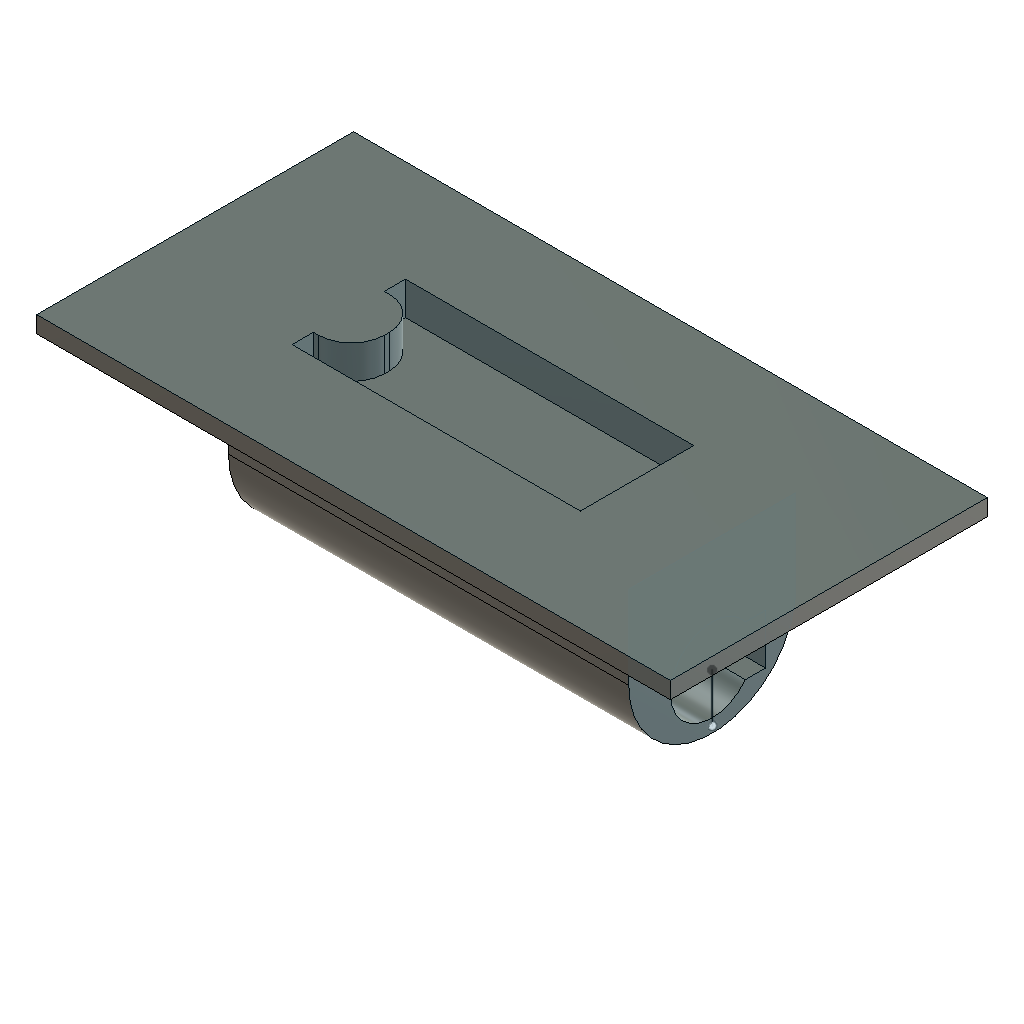
balancin (Ensamblaje) (Autodesk Fusion 360 archive; units mm, degrees)
design "balancin"
part number: 2026-09-28-04-10-51-977
Autodesk Fusion 360 part; units mm, degrees
sketch "Boceto1" plane through (0, 0, 0) normal (0, 1, 0) x (1, 0, 0)
  line L0 (-30, 20) -> (160, 20)
  line L1 (160, 20) -> (160, -75)
  line L2 (160, -75) -> (-30, -75)
  line L3 (-30, -75) -> (-30, 20)
  dimension "d1" = 190
  dimension "d2" = 95
  constraint horizontal L0
  constraint vertical L1
  constraint horizontal L2
  constraint vertical L3
  measures "d1" distance of L0.start L0.end
  measures "d2" distance of L0.start L2.end
extrude "Extruir1" add sketch "Boceto1" along normal blind 5
sketch "Boceto2" plane through (0, 0, 0) normal (0, -1, 0) x (1, 0, 0)
  line L0 (160, 75) -> (-30, 75)
  line L1 (-30, 75) -> (-30, -20)
  line L2 (-30, -20) -> (160, -20)
  line L3 (160, -20) -> (160, 75)
  line L4 (-30, 27.5) -> (5, 27.5)
  line L5 (65, 52.5) -> (5, 52.5)
  line L6 (125, 27.5) -> (125, 2.5)
  line L7 (5, 52.5) -> (125, 52.5)
  line L8 (125, 52.5) -> (125, 2.5)
  line L9 (125, 2.5) -> (5, 2.5)
  line L10 (5, 2.5) -> (5, 52.5)
  point P0 (65, 27.5)
  dimension "d5" = 47.5
  dimension "d6" = 95
  dimension "d7" = 25
  dimension "d8" = 60
  dimension "d9" = 60
  dimension "d10" = 25
  constraint horizontal L7
  constraint vertical L8
  constraint horizontal L9
  constraint vertical L10
  constraint coincident L10 L4.end
  measures "d5" distance of L0.end L4.start
  measures "d6" distance of L4.start P0
  measures "d7" distance of L5.start P0
  measures "d8" distance of L5.start L5.end
  measures "d9" distance of L6.start P0
  measures "d10" distance of L6.start L6.end
extrude "Extruir2" add sketch "Boceto2" along normal blind 50 contours L5 L6 L7 L8 L9 L10
sketch "Boceto3" plane through (125, 0, 0) normal (1, 0, 0) x (0, 0, -1)
  line L0 (-2.5, 0) -> (-52.5, 0)
  line L1 (-52.5, 0) -> (-52.5, -50)
  line L2 (-52.5, -50) -> (-2.5, -50)
  line L3 (-2.5, -50) -> (-2.5, 0)
  line L4 (-52.5, -50) -> (-27.5, -50)
  line L5 (-27.5, -50) -> (-27.5, -46)
  circle A0 centre (-27.5, -33.525) radius 12.475
  dimension "d13" = 25
  dimension "d14" = 4
  dimension "d15" = 24.95
  constraint coincident L1.end L2.start
  constraint perpendicular L1 L4
  constraint perpendicular L4 L5
  constraint coincident L5.end A0
  measures "d13" distance of L1.end L4.end
  measures "d14" distance of L4.end L5.end
  measures "d15" diameter of A0
extrude "Extruir3" cut sketch "Boceto3" against normal blind 150 contours A0
sketch "Boceto4" plane through (125, 0, 0) normal (1, 0, 0) x (0, 0, -1)
  circle A0 centre (-27.5, -33.525) radius 12.475
  line L0 (-2.5, 0) -> (-52.5, 0)
  line L1 (-52.5, 0) -> (-52.5, -50)
  line L2 (-52.5, -50) -> (-2.5, -50)
  line L3 (-2.5, -50) -> (-2.5, 0)
  line L4 (-27.5, -33.525) -> (-18.5, -33.525)
  line L5 (-18.5, -33.525) -> (-18.5, -26.025)
  line L6 (-18.5, -26.025) -> (-11.5, -26.025)
  line L7 (-11.5, -26.025) -> (-11.5, -41.025)
  line L8 (-11.5, -41.025) -> (-18.5, -41.025)
  line L9 (-18.5, -41.025) -> (-18.5, -26.025)
  dimension "d18" = 9
  dimension "d19" = 7.5
  dimension "d20" = 7
  dimension "d21" = 15
  constraint coincident A0.centre L4.start
  constraint perpendicular L4 L5
  constraint horizontal L6
  constraint vertical L7
  constraint horizontal L8
  constraint vertical L9
  measures "d18" distance of A0.centre L4.end
  measures "d19" distance of L4.end L5.end
  measures "d20" distance of L5.end L6.end
  measures "d21" distance of L6.end L7.end
extrude "Extruir4" cut sketch "Boceto4" against normal blind 180 contours A0 L6 L7 L8
fillet "Empalme1" radius 25 2 edges at (65, -50, 2.5) (65, -50, 52.5)
sketch "Boceto5" plane through (0, 0, 0) normal (0, 0, 1) x (1, 0, 0)
  line L0 (64.5, -25) -> (64.5, -45)
  line L1 (68.5, -25) -> (68.5, -45)
  line L2 (65.5, -25) -> (65.5, -5)
  line L3 (64.5, -5) -> (64.5, -25)
  line L4 (64.5, -45) -> (54.5, -45)
  line L5 (54.5, -45) -> (64.5, -45)
  line L6 (64.5, -45) -> (64.5, -5)
  line L7 (64.5, -5) -> (54.5, -5)
  line L8 (54.5, -5) -> (54.5, -45)
  line L9 (68.5, -45) -> (75.5, -45)
  line L10 (75.5, -45) -> (65.5, -45)
  line L11 (65.5, -45) -> (65.5, -5)
  line L12 (65.5, -5) -> (75.5, -5)
  line L13 (75.5, -5) -> (75.5, -45)
  line L14 (54.5, -40.8747) -> (75.5, -40.8747)
  line L15 (54.5, -23.0491) -> (75.5, -23.0491)
  dimension "d33" = 20
  dimension "d35" = 20
  dimension "d36" = 10
  dimension "d37" = 7
  dimension "d38" = 10
  constraint vertical L2
  constraint vertical L3
  constraint perpendicular L0 L4
  constraint horizontal L5
  constraint vertical L6
  constraint horizontal L7
  constraint vertical L8
  constraint perpendicular L1 L9
  constraint horizontal L10
  constraint vertical L11
  constraint horizontal L12
  constraint vertical L13
  constraint coincident L8 L14.start
  constraint coincident L13 L14.end
  constraint perpendicular L13 L14
  constraint coincident L8 L15.start
  constraint coincident L13 L15.end
  constraint perpendicular L13 L15
  measures "d33" distance of L0.start L0.end
  measures "d35" distance of L0.start L3.start
  measures "d36" distance of L0.end L4.end
  measures "d37" distance of L1.end L9.end
  measures "d38" distance of L2.end L12.end
extrude "Extruir5" cut sketch "Boceto5" along normal blind 31 contours L0 L3 L6 L8 L14 L15 | L2 L11 L13 L14 L15
sketch "Boceto6" plane through (0, 0, 11.5) normal (0, 0, 1) x (1, 0, 0)
  line L0 (54.5, -40.8747) -> (54.5, -26.025)
  line L1 (54.5, -26.025) -> (5, -26.025)
  line L2 (5, -26.025) -> (5, -41.025)
  line L3 (5, -41.025) -> (125, -41.025)
  line L4 (125, -41.025) -> (125, -26.025)
  line L5 (125, -26.025) -> (75.5, -26.025)
  line L6 (75.5, -26.025) -> (75.5, -40.8747)
  line L7 (75.5, -40.8747) -> (65.5, -40.8747)
  line L8 (65.5, -40.8747) -> (65.5, -26.025)
  line L9 (65.5, -26.025) -> (64.5, -26.025)
  line L10 (64.5, -26.025) -> (64.5, -40.8747)
  line L11 (64.5, -40.8747) -> (54.5, -40.8747)
  line L12 (64.5, -48.0409) -> (65.5441, -48.0409)
  line L13 (65.5441, -48.0409) -> (65.5441, -10.5894)
  line L14 (65.5441, -10.5894) -> (64.5, -10.5894)
  line L15 (64.5, -10.5894) -> (64.5, -48.0409)
  constraint horizontal L12
  constraint vertical L13
  constraint horizontal L14
  constraint vertical L15
extrude "Extruir6" add sketch "Boceto6" along normal blind 30 contours L3 L7 L8 L9 L10 L13 L15 | L7 L8 L9 L13 L14 L15 | L3 L12 L13 L15
sketch "Boceto7" plane through (65.5441, 0, 0) normal (1, 0, 0) x (0, 0, -1)
  arc A0 (-17.7987, -48.0409) -> (-11.5, -44.2094) centre (-27.5, -25) ccw
  line L0 (-17.7987, -48.0409) -> (-11.5, -48.0409)
  line L1 (-11.5, -48.0409) -> (-11.5, -44.2094)
  arc A1 (-41.5, -45.7123) -> (-37.2013, -48.0409) centre (-27.5, -25) ccw
  line L2 (-41.5, -45.7123) -> (-41.5, -48.0409)
  line L3 (-41.5, -48.0409) -> (-37.2013, -48.0409)
extrude "Extruir7" cut sketch "Boceto7" against normal blind 9
sketch "Boceto8" plane through (125, 0, 0) normal (1, 0, 0) x (0, 0, -1)
  line L0 (-11.5, -41.025) -> (-17.5313, -41.025)
  arc A0 (-17.5313, -26.025) -> (-17.5313, -41.025) centre (-27.5, -33.525) ccw
  line L1 (-17.5313, -26.025) -> (-11.5, -26.025)
  line L2 (-11.5, -26.025) -> (-11.5, -41.025)
  arc A1 (-52.5, -25) -> (-2.5, -25) centre (-27.5, -25) ccw
  line L3 (-2.5, -25) -> (-2.5, 0)
  line L4 (-2.5, 0) -> (-52.5, 0)
  line L5 (-52.5, 0) -> (-52.5, -25)
  line L6 (-27.5, -33.525) -> (-27.5, -48)
  constraint coincident A0.centre L6.start
  constraint vertical L6
sketch "Boceto9" plane through (0, 5, 0) normal (0, 1, 0) x (-1, 0, 0)
  line L0 (30, 75) -> (-160, 75)
  line L1 (-160, 75) -> (-160, -20)
  line L2 (-160, -20) -> (30, -20)
  line L3 (30, -20) -> (30, 75)
  line L4 (30, 75) -> (30, 27.5)
  line L5 (30, 27.5) -> (-65, 27.5)
  line L6 (-65, 27.5) -> (-102.5, 27.5)
  line L7 (-102.5, 27.5) -> (-102.5, 44.5)
  line L8 (-102.5, 44.5) -> (-27.5, 44.5)
  line L9 (-27.5, 44.5) -> (-27.5, 10.5)
  line L10 (-27.5, 10.5) -> (-102.5, 10.5)
  line L11 (-102.5, 10.5) -> (-102.5, 44.5)
  dimension "d47" = 47.5
  dimension "d48" = 95
  dimension "d49" = 37.5
  dimension "d50" = 17
  dimension "d51" = 34
  dimension "d52" = 75
  constraint coincident L0.start L3.end
  constraint perpendicular L0 L4
  constraint perpendicular L4 L5
  constraint parallel L5 L6
  constraint perpendicular L6 L7
  constraint horizontal L8
  constraint vertical L9
  constraint horizontal L10
  constraint vertical L11
  measures "d47" distance of L0.start L4.end
  measures "d48" distance of L4.end L5.end
  measures "d49" distance of L5.end L6.end
  measures "d50" distance of L6.end L7.end
  measures "d51" distance of L7.end L10.end
  measures "d52" distance of L7.end L8.end
extrude "Extruir8" cut sketch "Boceto9" against normal blind 10 contours L5 L6 L9 L10 L11 | L5 L6 L7 L8 L9 L11
sketch "Boceto10" plane through (0, 5, 0) normal (0, 1, 0) x (-1, 0, 0)
  line L0 (-27.5, 44.5) -> (-27.5, 10.5)
  line L1 (-27.5, 10.5) -> (-102.5, 10.5)
  line L2 (-102.5, 10.5) -> (-102.5, 44.5)
  line L3 (-102.5, 44.5) -> (-27.5, 44.5)
  line L4 (30, 75) -> (-160, 75)
  line L5 (-160, 75) -> (-160, -20)
  line L6 (-160, -20) -> (30, -20)
  line L7 (30, -20) -> (30, 75)
  line L8 (-27.5, 44.5) -> (-16.0562, 44.5)
  line L9 (-16.0562, 44.5) -> (-16.0562, 38.0888)
  line L10 (-16.0562, 38.0888) -> (-27.5, 38.0888)
  line L11 (-27.5, 38.0888) -> (-27.5, 44.5)
  line L12 (-27.5, 10.5) -> (-16.0562, 10.5)
  line L13 (-16.0562, 10.5) -> (-16.0562, 16.8458)
  line L14 (-16.0562, 16.8458) -> (-27.5, 16.8458)
  line L15 (-27.5, 16.8458) -> (-27.5, 10.5)
  constraint horizontal L8
  constraint vertical L9
  constraint horizontal L10
  constraint vertical L11
  constraint coincident L0.start L3.end
  constraint horizontal L12
  constraint vertical L13
  constraint horizontal L14
  constraint vertical L15
  constraint coincident L0.end L1.start
extrude "Extruir9" cut sketch "Boceto10" against normal blind 10 contours L0 L8 L9 L10 L11 | L0 L12 L13 L14 L15
fillet "Empalme2" radius 10 2 edges at (27.5, 0, 16.8458) (27.5, 0, 38.0888)
sketch "Boceto11" plane through (0, 5, 0) normal (0, 1, 0) x (-1, 0, 0)
  arc A0 (-17.5, 38.0888) -> (-27.5, 28.0888) centre (-17.5, 28.0888) ccw
  line L0 (-27.5, 28.0888) -> (-27.5, 26.8458)
  arc A1 (-27.5, 26.8458) -> (-17.5, 16.8458) centre (-17.5, 26.8458) ccw
  line L1 (-17.5, 16.8458) -> (-16.0562, 16.8458)
  line L2 (-16.0562, 16.8458) -> (-16.0562, 10.5)
  line L3 (-16.0562, 10.5) -> (-102.5, 10.5)
  line L4 (-102.5, 10.5) -> (-102.5, 44.5)
  line L5 (-102.5, 44.5) -> (-16.0562, 44.5)
  line L6 (-16.0562, 44.5) -> (-16.0562, 38.0888)
  line L7 (-16.0562, 38.0888) -> (-17.5, 38.0888)
  line L8 (30, 75) -> (-160, 75)
  line L9 (-160, 75) -> (-160, -20)
  line L10 (-160, -20) -> (30, -20)
  line L11 (30, -20) -> (30, 75)
